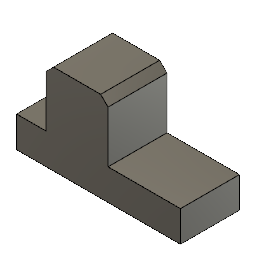
stepper_support_bumper v6 (Autodesk Fusion 360 design; units mm, degrees)
Autodesk Fusion 360 part; units mm, degrees
sketch "Sketch2" plane through (0, 0, 0) normal (0, 1, 0) x (1, 0, 0)
  line L0 (0, 4) -> (18.2, 4)
  line L1 (18.2, 4) -> (18.2, -4)
  line L2 (18.2, -4) -> (0, -4)
  line L3 (0, -4) -> (0, 4)
  line L4 (8.4, 4) -> (8.4, -4)
  line L5 (0, 0) -> (8.4, 0) construction
  line L6 (4.2, 4) -> (4.2, -4) construction
  line L7 (0, 4) -> (-4, 4)
  line L8 (-4, 4) -> (-4, -4)
  line L9 (-4, -4) -> (0, -4)
  line L10 (0, -4) -> (0, 4)
  point P0 (4.2, 0)
  dimension "d5" = 8
  dimension "d6" = 8.4
  dimension "d7" = 14
  dimension "d14" = 4
  dimension "d15" = 9.8
  constraint horizontal L0
  constraint vertical L1
  constraint horizontal L2
  constraint vertical L3
  constraint midpoint L5.start L3
  constraint coincident L0 L4.start
  constraint coincident L2 L4.end
  constraint perpendicular L2 L4
  constraint coincident L5.start origin
  constraint midpoint L4 L5.end
  constraint midpoint L5 P0
  constraint coincident L0 L6.start
  constraint coincident L2 L6.end
  constraint perpendicular L2 L6
  constraint coincident P0 L6
  constraint horizontal L7
  constraint vertical L8
  constraint horizontal L9
  constraint vertical L10
  constraint collinear L2 L9
  measures "d5" distance of L0.start L2.end
  measures "d6" distance of L3 L4
  measures "d7" distance of L1 L6
  measures "d14" distance of L8 L10
  measures "d15" distance of L1 L4
extrude "Extrude2" add sketch "Sketch2" along normal blind 8 contours L0 L2 L3 L4 L10
extrude "Extrude3" add sketch "Sketch2" against normal blind 4.2
chamfer "Chamfer1" distance 1 angle 45 2 edges at (0, 8, 0) (8.4, 8, 0)
sketch "Sketch1" plane through (0, 0, 0) normal (0, 1, 0) x (1, 0, 0)
  line L0 (3, -2.5) -> (-3, -2.5)
  line L1 (-3, -2.5) -> (-3, 2.5)
  line L2 (-3, 2.5) -> (3, 2.5)
  line L3 (3, 2.5) -> (3, -2.5)
  line L4 (3, -2.5) -> (-3, 2.5) construction
  line L5 (-3, -2.5) -> (3, 2.5) construction
  dimension "d1" = 5
  dimension "d2" = 6
  constraint perpendicular L0 L1
  constraint parallel L0 L2
  constraint parallel L1 L3
  constraint horizontal L0
  constraint coincident L4 origin
  constraint coincident L5 origin
  measures "d1" distance of L0.start L2.end
  measures "d2" distance of L0.start L0.end
extrude "Extrude1" [suppressed]
